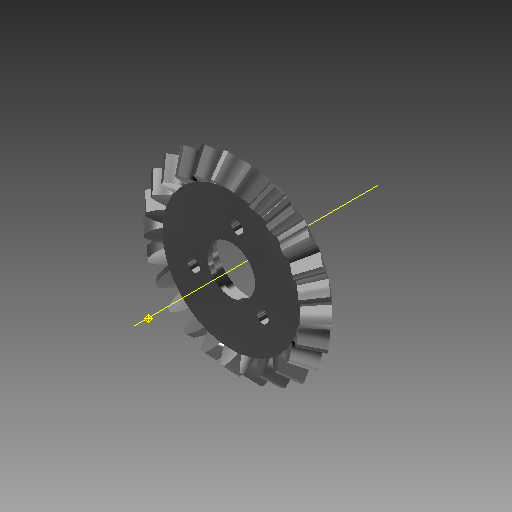
# Autodesk Inventor part: Kegelrad2
Saved by Autodesk Inventor 2018 (Build 220112000, 112)
## iProperties
Created: 2017-04-26
Part Number: Kegelrad2
Material: Siliziumnitrid
Document SubType Name: Modeling
Designer: Jochen Alt
Categories: <?xml version="1.0" encoding="UTF-16"?> <MemberInstance><Categories><FamilyTemplate><FamilyTemplateParameter ValueType="xs:double" Id="1" ObjectReferenceKey="da_z" ObjectType="kUserParameterObject"/><FamilyTemplateParameter ValueType="xs:double" Id="2" ObjectReferenceKey="da_b" ObjectType="kUserParameterObject"/><FamilyTemplateParameter ValueType="xs:double" Id="3" ObjectReferenceKey="da_beta" ObjectType="kUserParameterObject"/><FamilyTemplateParameter ValueType="xs:double" Id="4" ObjectReferenceKey="da_dae" ObjectType="kUserParameterObject"/><FamilyTemplateParameter ValueType="xs:double" Id="5" ObjectReferenceKey="da_ve" ObjectType="kUserParameterObject"/><FamilyTemplateParameter ValueType="xs:double" Id="6" ObjectReferenceKey="da_omega" ObjectType="kUserParameterObject"/><FamilyTemplateParameter ValueType="xs:string" Id="7" ObjectReferenceKey="EAIAABAAAAAAHwAAAAAAAIAAAAAAAAAA" ObjectType="83914240" SubObjectId="SurfaceGeometry"/></FamilyTemplate><ParamToTemplateMap><ParamToTemplate CategoryParameter="//CategoryParameter[@InternalName='046C89C9-8512-4d59-83FE-43B91F4F132A']" TemplateParameter="1"/><ParamToTemplate CategoryParameter="//CategoryParameter[@InternalName='2552DF32-E462-4b46-AEBF-C6C7768E72AC']" TemplateParameter="2"/><ParamToTemplate CategoryParameter="//CategoryParameter[@InternalName='C9EE641D-15FC-4fae-A226-E94C4372FDD7']" TemplateParameter="3"/><ParamToTemplate><ParamToTemplate CategoryParameter="//CategoryParameter[@InternalName='00B6519A-459B-49c7-AD84-2E56D39A5744']" ConstantValue="-0.000000"/></ParamToTemplate><ParamToTemplate><ParamToTemplate CategoryParameter="//CategoryParameter[@InternalName='04B31F0E-C7A6-4894-AA32-9629BEFACF47']" ConstantValue="1.000000"/></ParamToTemplate><ParamToTemplate><ParamToTemplate CategoryParameter="//CategoryParameter[@InternalName='43CBEC2E-7847-49e7-A936-2F7889FCB2D9']" ConstantValue="0.200000"/></ParamToTemplate><ParamToTemplate><ParamToTemplate CategoryParameter="//CategoryParameter[@InternalName='B1EFC894-105D-4ebd-86BF-FA20ED196853']" ConstantValue="0.266800"/></ParamToTemplate><ParamToTemplate><ParamToTemplate CategoryParameter="//CategoryParameter[@InternalName='51175063-3D10-4879-93E8-6246FE8B403D']" ConstantValue="2060000000.000000"/></ParamToTemplate><ParamToTemplate><ParamToTemplate CategoryParameter="//CategoryParameter[@InternalName='A3A52E27-4454-46a9-B0BD-C932399B70AF']" ConstantValue="0.300000"/></ParamToTemplate><ParamToTemplate CategoryParameter="//CategoryParameter[@InternalName='2A200944-5A8C-41ca-B96E-8520D2E510F1']" TemplateParameter="4"/><ParamToTemplate><ParamToTemplate CategoryParameter="//CategoryParameter[@InternalName='1A637F62-92C8-44bc-B81F-10802510B579']" ConstantValue="2.718746"/></ParamToTemplate><ParamToTemplate CategoryParameter="//CategoryParameter[@InternalName='B52DD4BE-6863-48fb-BF58-89EF6F9EC65C']" TemplateParameter="5"/><ParamToTemplate><ParamToTemplate CategoryParameter="//CategoryParameter[@InternalName='3956BFF2-84D2-457d-93C2-9B0613DEBA67']" ConstantValue="1.265401"/></ParamToTemplate><ParamToTemplate CategoryParameter="//CategoryParameter[@InternalName='739CFA02-461B-4bf8-8049-181FCAD8B28F']" TemplateParameter="6"/><ParamToTemplate><ParamToTemplate CategoryParameter="//CategoryParameter[@InternalName='A27E999F-E2CE-4481-8A2A-EBF499C4C3C5']" ConstantValue="-0.000000"/></ParamToTemplate><ParamToTemplate><ParamToTemplate CategoryParameter="//CategoryParameter[@InternalName='9E1B4470-B2D3-4ff1-B813-535BB4CDF51A']" ConstantValue="3520000.000000"/></ParamToTemplate><ParamToTemplate><ParamToTemplate CategoryParameter="//CategoryParameter[@InternalName='F8452263-BFF6-458c-9FB1-07C4B99E95CD']" ConstantValue="11400000.000000"/></ParamToTemplate><ParamToTemplate><ParamToTemplate CategoryParameter="//CategoryParameter[@InternalName='3E3BB259-FD49-497f-8171-6EBC954A3479']" ConstantValue="2.000000"/></ParamToTemplate><ParamToTemplate CategoryParameter="//CategoryParameter[@InternalName='27C3BAF2-7550-4e4b-AE2C-0DB134B7D9B7']" TemplateParameter="7"/></ParamToTemplateMap><Category DisplayName="Gear" InternalName="DC85795E-93AB-48d5-8EEE-5A27447B64BD" Mnemonic="Gear"><CategoryParameter DisplayName="z" InternalName="046C89C9-8512-4d59-83FE-43B91F4F132A" Mnemonic="z"/><CategoryParameter DisplayName="b" InternalName="2552DF32-E462-4b46-AEBF-C6C7768E72AC" Mnemonic="b"/><CategoryParameter DisplayName="||b|" InternalName="C9EE641D-15FC-4fae-A226-E94C4372FDD7" Mnemonic="beta"/><CategoryParameter DisplayName="x" InternalName="00B6519A-459B-49c7-AD84-2E56D39A5744" Mnemonic="x"/><CategoryParameter DisplayName="a*" InternalName="04B31F0E-C7A6-4894-AA32-9629BEFACF47" Mnemonic="a"/><CategoryParameter DisplayName="c*" InternalName="43CBEC2E-7847-49e7-A936-2F7889FCB2D9" Mnemonic="c"/><CategoryParameter DisplayName="r|.f|*" InternalName="B1EFC894-105D-4ebd-86BF-FA20ED196853" Mnemonic="rf"/><CategoryParameter DisplayName="E" InternalName="51175063-3D10-4879-93E8-6246FE8B403D" Mnemonic="E"/><CategoryParameter DisplayName="||m|" InternalName="A3A52E27-4454-46a9-B0BD-C932399B70AF" Mnemonic="mi"/><Category DisplayName="BevelGear" InternalName="0C98F69A-0C2B-4791-B2FE-7691BB227E77" Mnemonic="BevelGear"><CategoryParameter DisplayName="d|.ae|" InternalName="2A200944-5A8C-41ca-B96E-8520D2E510F1" Mnemonic="dae"/><CategoryParameter DisplayName="d|.ai|" InternalName="1A637F62-92C8-44bc-B81F-10802510B579" Mnemonic="dai"/><CategoryParameter DisplayName="A|.e|" InternalName="B52DD4BE-6863-48fb-BF58-89EF6F9EC65C" Mnemonic="ve"/><CategoryParameter DisplayName="A|.i|" InternalName="3956BFF2-84D2-457d-93C2-9B0613DEBA67" Mnemonic="vi"/><CategoryParameter DisplayName="||S|" InternalName="739CFA02-461B-4bf8-8049-181FCAD8B28F" Mnemonic="omega"/><CategoryParameter DisplayName="x|.t|" InternalName="A27E999F-E2CE-4481-8A2A-EBF499C4C3C5" Mnemonic="xt"/><CategoryParameter DisplayName="||s||.Flim|" InternalName="9E1B4470-B2D3-4ff1-B813-535BB4CDF51A" Mnemonic="sFlim"/><CategoryParameter DisplayName="||s||.Hlim|" InternalName="F8452263-BFF6-458c-9FB1-07C4B99E95CD" Mnemonic="sHlim"/><CategoryParameter DisplayName="Typ" InternalName="3E3BB259-FD49-497f-8171-6EBC954A3479" Mnemonic="type"/><CategoryParameter DisplayName="PitchDiameter" InternalName="27C3BAF2-7550-4e4b-AE2C-0DB134B7D9B7" Mnemonic="IDS_PITCHDIAM"/></Category></Category></Categories></MemberInstance>
Mass: 5.89525 g
Surface Area: 20.5656 cm^2
Volume: 1.85385 cm^3
Density: 3.18 g/cm^3
Appearance: Chrom - poliert - schwarz
CustomPartVersion: 1
Author: Jochen Alt
Autodesk Inventor part; units mm, degrees
ref_plane "Netzebene2" through (0, 0, 0) normal (0.9921147, 0.1253332, 0) x (0, 0, 1)
sketch "Skizze des Zahnradkörpers" plane through (0, 0, 0) normal (1, 0, 0) x (0, 1, 0)
  line L0 (0, 0) -> (14.5438, -17.2897) construction
  line L1 (14.5438, -17.2897) -> (16.526, -15.3836)
  line L2 (16.526, -15.3836) -> (0, 0) construction
  line L3 (15.625, -16.25) -> (0, 0) construction
  line L4 (11.9632, -14.2219) -> (13.5937, -12.654)
  line L5 (14.5438, -17.2897) -> (11.9632, -14.2219)
  line L6 (16.526, -15.3836) -> (13.5937, -12.654)
  line L7 (0, -20.7476) -> (0, 3.4579) projected
  line L8 (0, -16.25) -> (16.526, -16.25) construction
  dimension "d0" = 31.25
  dimension "d1" = 29.0875
  dimension "d2" = 33.0521
  dimension "d3" = 4
  dimension "d4" = 15.3836
  constraints: 16 end point, 4 point on line, 3 perpendicular, 2 collinear, 1 horizontal alignment, 1 vertical alignment
  measures "d0" diameter of L3.start L7
  measures "d1" diameter of L0.end L7
  measures "d2" diameter of L1.end L7
  measures "d3" distance between parallel lines of L1 L4
  measures "d4" vertical distance of L1.end L0.start
revolve "Zahnradkörper" add sketch "Skizze des Zahnradkörpers" angle 360 about axis through (0, 0, 0) along (0, 0, 1)
ref_plane "Zahnebene" through (0, 15.625, -16.25) normal (0, -0.6931087, 0.7208331) x (1, 0, 0)
sketch "Startskizze" plane through (0, 15.625, -16.25) normal (0, -0.6931087, 0.7208331) x (1, 0, 0)
  line L0 (0, -26.427) -> (0, 6.8277) projected
  arc A0 (-0.2859, -1.83) -> (-2.3519, 1.9583) centre (-9.4505, -4.3707) ccw
  arc A1 (2.3519, 1.9583) -> (0.2859, -1.83) centre (9.4505, -4.3707) ccw
  line L1 (-0.2859, -1.83) -> (0.2859, -1.83)
  arc A2 (2.3519, 1.9583) -> (-2.3519, 1.9583) centre (0, -21.6763) ccw
  dimension "d7" = 9.5103
  dimension "d8" = 9.4505
  dimension "d9" = 17.3057
  dimension "d57" = 23.7513
  dimension "d58" = 19.8463
  constraints: 6 point on circle, 3 centre point, 3 symmetric about line, 2 end point, 1 coincident, 1 perpendicular, 1 other
  measures "d7" radius of A0
  measures "d8" horizontal distance of point (0, -21.676) A0.centre
  measures "d9" vertical distance of point (0, -21.676) A0.centre
  measures "d57" radius of A2
  measures "d58" distance from line of A2.centre L1
ref_plane "Endebene" through (0, 12.7573, -13.2676) normal (0, -0.6931087, 0.7208331) x (1, 0, 0)
sketch "Endskizze" plane through (0, 12.7573, -13.2676) normal (0, -0.6931087, 0.7208331) x (1, 0, 0)
  line L0 (0, -20.4092) -> (0, 5.3002) projected
  arc A0 (-0.2337, -1.4743) -> (-1.9226, 1.6225) centre (-7.7255, -3.5512) ccw
  arc A1 (1.9226, 1.6225) -> (0.2337, -1.4743) centre (7.7255, -3.5512) ccw
  line L1 (-0.2337, -1.4743) -> (0.2337, -1.4743)
  arc A2 (1.9226, 1.6225) -> (-1.9226, 1.6225) centre (0, -17.6979) ccw
  dimension "d12" = 7.7743
  dimension "d15" = 7.7255
  dimension "d16" = 14.1468
  dimension "d59" = 19.4159
  dimension "d60" = 16.2237
  constraints: 6 point on circle, 3 centre point, 3 symmetric about line, 2 end point, 1 coincident, 1 other
  measures "d12" radius of A0
  measures "d15" horizontal distance of A0.centre point (0, -17.698)
  measures "d16" vertical distance of A0.centre point (0, -17.698)
  measures "d59" radius of A2
  measures "d60" distance from line of A2.centre L1
loft "Loft" cut profiles "Startskizze", "Endskizze"
pattern_circular "Circular Pattern" count 25 over 360 about axis through (0, 0, 0) along (0, 0, 1) of "Loft"
sketch3d "3D-Skizze rechts"
ref_plane "Endebene rechts" through (-1.4136, 12.6787, -13.2676) normal (0.076804, -0.6888402, 0.7208331) x (0.9938415, 0.1108109, 0)
sketch "Endskizze rechts" plane through (-1.4136, 12.6787, -13.2676) normal (0.076804, -0.6888402, 0.7208331) x (0.9938415, 0.1108109, 0)
  arc A0 (-0.2337, -1.4743) -> (-1.9226, 1.6225) centre (-7.7255, -3.5512) ccw
  line L0 (0, -23.187) -> (0, 7.1165) projected
  arc A1 (1.9226, 1.6225) -> (0.2337, -1.4743) centre (7.7255, -3.5512) ccw
  line L1 (-0.2337, -1.4743) -> (0.2337, -1.4743)
  arc A2 (1.9226, 1.6225) -> (-1.9226, 1.6225) centre (0, -17.6979) ccw
  dimension "d70" = 7.7255
  dimension "d71" = 14.1468
  dimension "d72" = 7.7743
  dimension "d73" = 16.2237
  dimension "d74" = 19.4159
  constraints: 6 point on circle, 3 centre point, 3 symmetric about line, 2 end point, 1 coincident, 1 perpendicular, 1 other
  measures "d70" horizontal distance of A2.centre A0.centre
  measures "d71" vertical distance of point (0, -17.698) A0.centre
  measures "d72" radius of A0
  measures "d73" distance from line of point (0, -17.698) L1
  measures "d74" radius of A2
feature "Erhebung rechts" [suppressed]
pattern_circular "Runde Anordnung rechts" [suppressed]
sketch3d "3D-Skizze links"
ref_plane "Endebene links" through (1.437, 12.6787, -13.2788) normal (-0.0780335, -0.6884703, 0.7210544) x (0.9936379, -0.1126222, 0)
sketch "Endskizze links" plane through (1.437, 12.6787, -13.2788) normal (-0.0780335, -0.6884703, 0.7210544) x (0.9936379, -0.1126222, 0)
  line L0 (0, -24.4626) -> (0, 8.4031) projected
  arc A0 (-0.2337, -1.4684) -> (-1.9226, 1.6284) centre (-7.7255, -3.5453) ccw
  arc A1 (1.9226, 1.6284) -> (0.2337, -1.4684) centre (7.7255, -3.5453) ccw
  line L1 (-0.2337, -1.4684) -> (0.2337, -1.4684)
  ellipse E0 centre (0, -8.7677) end of major axis (13.5937, -8.7677) minor radius 9.8018 projected
  arc A2 (1.9226, 1.6284) -> (-1.9226, 1.6284) centre (0, -17.6921) ccw
  dimension "d56" = 9.8018
  dimension "d30" = 7.7743
  dimension "d31" = 7.7255
  dimension "d32" = 14.1468
  dimension "d61" = 19.4159
  dimension "d62" = 16.2237
  constraints: 6 point on circle, 3 centre point, 3 symmetric about line, 2 end point, 1 coincident, 2 other
  measures "d30" radius of A0
  measures "d31" horizontal distance of point (0, -17.692) A0.centre
  measures "d32" vertical distance of A0.centre point (0, -17.692)
  measures "d61" radius of A2
  measures "d62" distance from line of point (0, -17.692) L1
feature "Erhebung links" [suppressed]
pattern_circular "Runde Anordnung links" [suppressed]
sketch "Körperskizze" plane through (0, 0, 0) normal (1, 0, 0) x (0, 1, 0)
  line L0 (0, -18.0566) -> (0, -12.688) projected
  line L1 (14.5438, -17.2897) -> (11.9632, -14.2219) projected
  line L2 (11.9632, -14.2219) -> (0, -14.2219)
  line L3 (14.5438, -17.2897) -> (0, -17.2897)
  constraints: 4 end point, 2 perpendicular, 2 point on line
revolve "Festkörper" add sketch "Körperskizze" angle 360 about axis through (0, 0, 0) along (0, 0, 1)
sketch "Sketch6" plane through (0, 0, 0) normal (1, 0, 0) x (0, 1, 0)
  line L0 (15.625, -16.25) -> (0, 0) projected
  line L1 (0, -19.5) -> (0, 3.25) projected
surface revolve "Flankendurchmesser" sketch "Sketch6" angle 360 about axis through (0, 0, 0) along (0, 0, 1) shown no curves L0
sketch "Skizze8" plane through (0, 0, -14.2219) normal (0, 0, 1) x (1, 0, 0)
  circle A0 centre (5.4907, -4.342) radius 1.05
  circle A1 centre (1.0149, 6.926) radius 1.05
  circle A2 centre (-6.5056, -2.5841) radius 1.05
  point P0 (0, 0)
  dimension "d99" = 360
  constraints: 3 centre point, 7 other
extrude "Extrusion1" cut sketch "Skizze8" against normal through all
sketch "Skizze9" plane through (0, 0, -17.2897) normal (0, 0, -1) x (-1, 0, 0)
  arc A0 (3.2451, 14.1771) -> (0.3825, 14.5387) centre (0, 0) ccw projected
  circle A1 centre (0, 0) radius 5.6
  dimension "d106" = 11.2
  constraints: 1 centre point, 1 coincident
  measures "d106" diameter of A1
extrude "Extrusion2" cut sketch "Skizze9" against normal blind 2.2
sketch "Skizze10" plane through (0, 0, -17.2897) normal (0, 0, -1) x (-1, 0, 0)
  arc A0 (3.2451, 14.1771) -> (0.3825, 14.5387) centre (0, 0) ccw projected
  circle A1 centre (0, 0) radius 4.15
  dimension "d109" = 8.3
  constraints: 1 centre point, 1 coincident
  measures "d109" diameter of A1
extrude "Extrusion3" cut sketch "Skizze10" against normal through all
equation "\"d0\" = da_de"
equation "\"d1\" = da_dfe"
equation "\"d2\" = da_dae"
equation "\"d3\" = da_b"
equation "\"d4\" = da_ve"
equation "\"d7\" = fd_rr"
equation "\"d8\" = fd_x"
equation "\"d9\" = fd_y"
equation "\"d57\" = 0.5 * fd_dva + 0.3 * da_he"
equation "\"d58\" = 0.5 * fd_dva - 1.12 * da_he"
equation "\"da_teethtype\" = 0"
equation "\"da_b\" = 4"
equation "\"da_de\" = 31.25"
equation "\"da_dae\" = 33.05208"
equation "\"da_dfe\" = 29.0875"
equation "\"da_le\" = 22.54336"
equation "\"da_omega\" = 90deg"
equation "\"da_beta\" = 0"
equation "\"da_delta\" = 43.876697deg"
equation "\"da_alpha\" = 25deg"
equation "\"da_he\" = 2.75"
equation "\"da_ve\" = 15.38361"
equation "\"da_zv\" = 34.682094"
equation "\"fd_loft\" = da_b + 0.05 * da_he"
equation "\"fd_x\" = fd_x1 + fd_x2"
equation "\"fd_y\" = fd_y1 - fd_y2"
equation "\"fd_dd\" = fd_dva - 0.8 * da_he"
equation "\"da_dvw\" = 43.35262"
equation "\"d11\" = fd_loft"
equation "\"da_dm\" = 28.47757"
equation "\"da_x\" = 0"
equation "\"da_m\" = 1.25"
equation "\"d50\" = da_omega"
equation "\"fd_rr\" = 9.510295"
equation "\"fd_dva\" = 45.852617"
equation "\"fd_x1\" = 0.992309"
equation "\"fd_x2\" = 8.458207"
equation "\"fd_y1\" = 21.653584"
equation "\"fd_y2\" = 4.347926"
body "Solid1"
body "Srf1"
